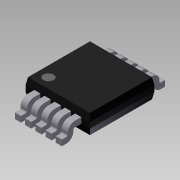
# Autodesk Inventor part: SOIC-10 micro (RM-10)
Saved by Autodesk Inventor 2011 (Build 150239000, 239)
## iProperties
Created: 2010-11-20
Part Number: SOIC-10 micro (RM-10)
Document SubType Name: Modeling
Designer: abbath
Density: 1 g/cm^3
Author: abbath
Autodesk Inventor part; units mm, degrees
ref_plane "YZ Plane" through (0, 0, 0) normal (1, 0, 0) x (0, 1, 0)
sketch "Эскиз1" plane through (0, 0, 0) normal (0, 0, 1) x (1, 0, 0)
  line L0 (-1.575, 1.575) -> (1.575, 1.575)
  line L1 (1.575, 1.575) -> (1.575, -1.575)
  line L2 (1.575, -1.575) -> (-1.575, -1.575)
  line L3 (-1.575, -1.575) -> (-1.575, 1.575)
  point P0 (0, 0)
  dimension "d0" = 1.575
  dimension "d1" = 1.575
  dimension "d2" = 3.15
  dimension "d3" = 3.15
  constraints: 8 end point, 2 parallel, 1 horizontal, 1 perpendicular
  measures "d0" distance from line of L3 point (0, 0)
  measures "d1" distance from line of L0 point (0, 0)
  measures "d2" distance between parallel lines of L2 L0
  measures "d3" distance between parallel lines of L1 L3
extrude "Выдавливание1" add sketch "Эскиз1" along normal blind 1.09
sketch "Эскиз2" plane through (1.575, -1.575, 0) normal (1, 0, 0) x (0, 0, -1)
  line L0 (-1.09, 3.15) -> (-1.09, 0) projected
  line L1 (0, 0) -> (-1.09, 0) projected
  line L2 (0, 3.15) -> (0, 0) projected
  line L3 (0, 3.15) -> (-1.09, 3.15) projected
  line L4 (-0.76, 0) -> (-0.76, 3.15)
  line L5 (-0.48, 0) -> (-0.48, 3.15)
  line L6 (-0.48, 0) -> (-0.15, 0.0582)
  line L7 (-0.15, 0.0582) -> (-0.15, 3.0918)
  line L8 (-0.15, 3.0918) -> (-0.48, 3.15)
  line L9 (-0.76, 3.15) -> (-1.09, 3.0918)
  line L10 (-0.76, 0) -> (-1.09, 0.0582)
  point P0 (0, 1.575)
  dimension "d6" = 0.28
  dimension "d7" = 0.15
  dimension "d8" = 0.33
  dimension "d9" = 0.33
  dimension "d10" = 10
  dimension "d11" = 10
  constraints: 14 end point, 6 point on line, 3 parallel, 2 perpendicular
  measures "d6" distance between parallel lines of L5 L4
  measures "d7" distance between parallel lines of L2 L7
  measures "d8" distance between parallel lines of L7 L5
  measures "d9" distance between parallel lines of L0 L4
  measures "d10" angle of L10 L1
  measures "d11" angle of L3 L9
extrude "Выдавливание2" cut sketch "Эскиз2" against normal through all contours L3 L9 L0 | L10 L1 L0 | L3 L2 L1 L6 L7 L8
sketch "Эскиз3" plane through (-1.575, -1.575, 0.48) normal (0, -1, 0) x (1, 0, 0)
  line L0 (0, 0.28) -> (0, 0.61) projected
  line L1 (3.15, 0.28) -> (0, 0.28) projected
  line L2 (3.15, 0.61) -> (3.15, 0.28) projected
  line L3 (0, 0.61) -> (3.15, 0.61) projected
  line L4 (0, -0.33) -> (0, 0) projected
  line L5 (3.15, -0.33) -> (0, -0.33) projected
  line L6 (3.15, 0) -> (3.15, -0.33) projected
  line L7 (0, 0) -> (3.15, 0) projected
  line L8 (0, 0.28) -> (0.0582, 0.61)
  line L9 (0, 0) -> (0.0582, -0.33)
  line L10 (3.15, 0) -> (3.0918, -0.33)
  line L11 (3.15, 0.28) -> (3.0918, 0.61)
  point P0 (1.575, -0.48)
  dimension "d14" = 10
  dimension "d15" = 10
  constraints: 8 end point, 4 point on line, 2 parallel
  measures "d14" angle of L8 L0
  measures "d15" angle of L11 L2
extrude "Выдавливание3" cut sketch "Эскиз3" against normal through all contours L0 L3 L8 | L11 L3 L2 | L4 L9 L5 | L6 L5 L10
ref_plane "РабПлоскость1" through (-1, -1.575, 0.76) normal (-1, 0, 0) x (0, 0, 1)
sketch "Эскиз4" plane through (-1, -1.575, 0.76) normal (-1, 0, 0) x (0, 0, 1)
  line L0 (0.33, 0.0582) -> (0, 0) projected
  line L1 (0.33, 3.0918) -> (0.33, 0.0582) projected
  line L2 (0, 3.15) -> (0.33, 3.0918) projected
  line L3 (0, 0) -> (0, 3.15) projected
  line L4 (0, 0) -> (0, 3.15) projected
  line L5 (-0.28, 3.15) -> (0, 3.15) projected
  line L6 (-0.28, 3.15) -> (-0.28, 0) projected
  line L7 (-0.28, 0) -> (0, 0) projected
  line L8 (-0.61, 3.0918) -> (-0.28, 3.15) projected
  line L9 (-0.61, 0.0582) -> (-0.61, 3.0918) projected
  line L10 (-0.28, 0) -> (-0.61, 0.0582) projected
  line L11 (-0.28, 3.15) -> (-0.28, 0) projected
  line L12 (0, -0.32) -> (0, 0)
  line L13 (0, 0) -> (-0.28, 0)
  line L14 (-0.28, 0) -> (-0.28, -0.32)
  line L15 (-0.76, 1.575) -> (0.8724, 1.575) construction
  line L16 (-0.48, -0.95) -> (-0.76, -0.95)
  line L17 (-0.76, -0.95) -> (-0.76, -0.74)
  line L18 (-0.48, -0.95) -> (-0.48, -0.74)
  line L19 (-0.35, -0.39) -> (-0.41, -0.39)
  line L20 (-0.35, -0.67) -> (-0.41, -0.67)
  arc A0 (-0.35, -0.39) -> (-0.28, -0.32) centre (-0.35, -0.32) ccw
  arc A1 (-0.41, -0.67) -> (-0.48, -0.74) centre (-0.41, -0.74) ccw
  arc A2 (-0.35, -0.67) -> (0, -0.32) centre (-0.35, -0.32) ccw
  arc A3 (-0.41, -0.39) -> (-0.76, -0.74) centre (-0.41, -0.74) ccw
  dimension "d19" = 2.525
  dimension "d20" = 0.15
  dimension "d21" = 0.28
  dimension "d22" = 0.28
  dimension "d23" = 0.56
  dimension "d24" = 0.28
  dimension "d25" = 0.14
  dimension "d26" = 0.14
  constraints: 18 end point, 8 point on circle, 6 tangent, 5 parallel, 4 centre point, 4 perpendicular, 3 collinear, 2 coincident
  measures "d19" distance between parallel lines of L16 L15
  measures "d20" distance between parallel lines of L17 L9
  measures "d21" distance between parallel lines of L14 L12
  measures "d22" distance between parallel lines of L18 L17
  measures "d23" distance between parallel lines of L19 L16
  measures "d24" distance between parallel lines of L20 L19
  measures "d25" diameter of A0
  measures "d26" diameter of A1
extrude "Выдавливание4" add sketch "Эскиз4" along normal mid plane 0.3 contours L12 A2 L20 A1 L18 L16 L17 A3 L19 A0 L14 L7
ref_plane "РабПлоскость2" through (-1.575, 0, 0.48) normal (0, 1, 0) x (1, 0, 0)
mirror "Зеркальное отражение1" about plane through (-1.575, 0, 0.48) normal (0, 1, 0) of "Выдавливание4"
pattern_linear "Прямоуг.массив1" count 5 spacing 0.5 along (1, 0, 0) of "Выдавливание4", "Зеркальное отражение1"
sketch "Эскиз5" plane through (0, 0, 1.09) normal (0, 0, 1) x (1, 0, 0)
  line L0 (-1.5168, 1.5168) -> (-1.5168, -1.5168) projected
  line L1 (-1.5168, -1.5168) -> (1.5168, -1.5168) projected
  circle A0 centre (-1.0168, -1.0168) radius 0.25
  point P0 (0, 0)
  dimension "d33" = 0.5
  dimension "d36" = 0.5
  dimension "d37" = 0.5
  constraints: 1 centre point
  measures "d33" diameter of A0
  measures "d36" distance from line of A0.centre L1
  measures "d37" distance from line of A0.centre L0
extrude "Выдавливание5" cut sketch "Эскиз5" against normal blind 0.01
equation "\"d0\" = 0.5 * d3"
equation "\"d1\" = 0.5 * d2"
equation "\"d8\" = d9"
equation "\"d22\" = d21"
equation "\"d24\" = d21"
equation "\"d25\" = 0.5 * d21"
equation "\"d26\" = 0.5 * d21"
equation "\"d36\" = d33"
equation "\"d37\" = d33"
